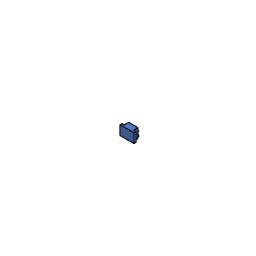
Taste_x1 (Autodesk Fusion 360 design; units mm, degrees)
Autodesk Fusion 360 part; units mm, degrees
sketch "Skizze1" plane through (0, 0, 59.536) normal (0, 0, -1) x (1, 0, 0)
  line L0 (54.288, -85.97) -> (62.288, -85.97)
  line L1 (62.288, -85.97) -> (62.288, -82.97)
  line L2 (62.288, -82.97) -> (54.288, -82.97)
  line L3 (54.288, -82.97) -> (54.288, -85.97)
  line L4 (64.188, -82.82) -> (62.188, -82.82)
  line L5 (62.188, -82.82) -> (62.188, -86.47)
  line L6 (62.188, -86.47) -> (54.388, -86.47)
  line L7 (54.388, -86.47) -> (54.388, -82.82)
  line L8 (54.388, -82.82) -> (52.388, -82.82)
  line L9 (52.388, -82.82) -> (52.388, -81.07)
  line L10 (52.388, -81.07) -> (64.188, -81.07)
  line L11 (64.188, -81.07) -> (64.188, -82.82)
  line L12 (50.288, -82.97) -> (50.288, -85.97)
  line L13 (40.65, -82.97) -> (67.1, -82.97)
  line L14 (-54.35, -82.97) -> (27.15, -82.97)
  line L15 (56.538, -80.97) -> (60.038, -80.97)
  point P0 (54.288, -85.97)
  point P1 (50.288, -85.97)
  dimension "d132_1_2_3" = 0.1
  dimension "d133_1_2_3" = 0.1
  dimension "d137_1_2_3" = 0.5
  dimension "d139_1_2_3" = 2
  dimension "d140_1_2_3" = 2
  dimension "d494" = 0.1
  dimension "d495" = 0.15
  constraint horizontal L4
  constraint perpendicular L0 L5
  constraint perpendicular L5 L6
  constraint perpendicular L0 L7
  constraint perpendicular L7 L8
  constraint perpendicular L0 L9
  constraint perpendicular L7 L10
  constraint perpendicular L10 L11
  constraint horizontal L4.end L7.end
  measures "d132_1_2_3" distance of L1 L5
  measures "d133_1_2_3" distance of L3 L7
  measures "d137_1_2_3" distance of L0 L6
  measures "d139_1_2_3" distance of L7.end L8.end
  measures "d140_1_2_3" distance of L4.start L4.end
  measures "d494" distance of L10 L15
  measures "d495" distance of L4 L13
extrude "Extrusion1" add sketch "Skizze1" along normal blind 7.8 contours L0 L2 L5 L7 L13 | L0 L5 L6 L7 | L2 L4 L5 L7 L8 L9 L10 L11 L13
sketch "Skizze2" plane through (0, 86.47, 0) normal (0, 1, 0) x (-1, 0, 0)
  line L0 (-54.388, 59.536) -> (-62.188, 59.536)
  line L1 (-62.188, 59.536) -> (-62.188, 51.736)
  line L2 (-62.188, 51.736) -> (-54.388, 51.736)
  line L3 (-54.388, 51.736) -> (-54.388, 59.536)
  line L4 (-62.0634, 52.736) -> (-54.5126, 52.736) construction
  line L5 (-54.5126, 52.736) -> (-54.5126, 60.336) construction
  line L6 (-54.5126, 60.336) -> (-62.0634, 60.336) construction
  line L7 (-62.0634, 60.336) -> (-62.0634, 52.736) construction
  point P0 (-58.288, 60.336)
  point P1 (-58.288, 59.536)
  dimension "d151_1_2_3" = 1
  dimension "d381_2_3" = 0.8
  text T0 "x1" font "Arial" height 7.6 bold align ink ink in box 0 x 0 at (-62.0534, 52.756) x (1, 0) y (0, 1) spacing 1 height is em
  constraint perpendicular L4 L5
  constraint parallel L4 L6
  constraint parallel L5 L7
  constraint midpoint L6 P0
  constraint midpoint L0 P1
  constraint vertical P0 P1
  measures "d151_1_2_3" distance of L2 L4
  measures "d381_2_3" distance of L0 L6
emboss "Prägen1" depth 1 profiles "Skizze2" section 1 text T0 onto face at (59.588, 86.47, 54.336)
move_body "Verschieben1" bodies 1 to x (1, 0, 0) y (0, 1, 0) z (0, 0, 1) at (0, 0, 0.2)
equation "d133_1_2_3 = d132_1_2_3"
equation "d139_1_2_3 = 4.00 mm / 2"
equation "d140_1_2_3 = d139_1_2_3"
